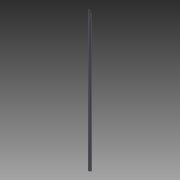
# Autodesk Inventor part: Needle3
Saved by Autodesk Inventor 2011 SP2 (Build 150309200, 309)
## iProperties
Created: 2011-01-21
Part Number: Needle3
Document SubType Name: Modeling
Designer: sungwook
Density: 7.75 g/cm^3
Material: Stainless Steel, 440C
Mass: 0.0578212 g
Surface Area: 1.01049 cm^2
Volume: 0.00746081 cm^3
Author: sungwook
Autodesk Inventor part; units mm, degrees
ref_plane "YZ Plane" through (0, 0, 0) normal (1, 0, 0) x (0, 1, 0)
ref_plane "XZ Plane" through (0, 0, 0) normal (0, 1, 0) x (-1, 0, 0)
ref_plane "UCS1: YZ Plane" through (-0.5, 0, 50) normal (0.9659, 0, 0.2588) x (0.2588, 0, -0.9659)
sketch "Sketch1" plane through (0, 0, 0) normal (0, 0, 1) x (1, 0, 0)
  circle A0 centre (0, 0) radius 0.5
  dimension "d0" = 1
  constraints: 1 centre point, 1 coincident
  measures "d0" diameter of A0
extrude "Extrusion1" add sketch "Sketch1" along normal blind 50
sketch "Sketch2" plane through (0, 0, 50) normal (0, 0, 1) x (1, 0, 0)
  circle A0 centre (0, 0) radius 0.5 projected
  line L0 (-0.7, 0) -> (0.7, 0) projected
  line L1 (0, -0.7) -> (0, 0.7) projected
  point P0 (0, 0.5)
  point P1 (0.5, 0)
  point P2 (-0.5, 0)
  constraints: 3 point on circle, 3 point on line
sketch "Sketch3" plane through (-0.5, 0, 50) normal (0, 1, 0) x (0.9659, 0, 0.2588)
  point P0 (0, 0)
sketch "Sketch4" plane through (0, 0, 0) normal (0, 1, 0) x (-1, 0, 0)
  line L0 (-0.5, 0) -> (-0.5, 50) projected
  line L1 (0.5, 0) -> (0.5, 50) projected
  line L2 (0.5, 50) -> (-0.5, 47.2525)
  line L3 (-0.5, 50) -> (0.5, 50) projected
  point P0 (0, 0)
  dimension "d9" = 70
  constraints: 2 end point, 1 point on line
  measures "d9" angle of L2 L3
extrude "Extrusion2" cut sketch "Sketch4" along normal through all both and the other way through all
sketch "Sketch5" plane through (0, 0, 0) normal (0, 0, -1) x (-1, 0, 0)
  circle A0 centre (0, 0) radius 0.5 projected
  circle A1 centre (0, 0) radius 0.35
  dimension "d12" = 0.7
  constraints: 1 centre point, 1 coincident
  measures "d12" diameter of A1
extrude "Hole" cut sketch "Sketch5" against normal through all contours A1
ref_plane "Work Plane1" through (0, 0, 30) normal (0, 0, 1) x (1, 0, 0)
sketch "Sketch6" plane through (0, 0, 30) normal (0, 0, 1) x (1, 0, 0)
  circle A0 centre (0, 0) radius 0.6
  dimension "d16" = 1.2
  constraints: 1 centre point, 1 coincident
  measures "d16" diameter of A0
extrude "Extrusion4" [suppressed]
body "Solid1"
